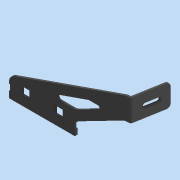
# Autodesk Inventor part: 0 零件
Saved by Autodesk Inventor 2020 (Build 240168000, 168)
## iProperties
Created: 2020-11-03
Part Number: 0 零件
Material: 鋼、碳鋼
Document SubType Name: Sheet Metal
Designer: p2013
Density: 7.85 g/cm^3
Appearance: 一般
Sheet Metal Rule: 預設 mm (_M)
Flat Pattern Width: 7.87536 cm
Flat Pattern Length: 32.1122 cm
Flat Pattern Area: 252.896 cm^2
Sheet Metal Width: 78.754 mm
Sheet Metal Length: 321.122 mm
Sheet Metal Area: 25289.554 mm^2
Author: p2013
Autodesk Inventor part; units mm, degrees
ref_plane "YZ Plane" through (0, 0, 0) normal (1, 0, 0) x (0, 1, 0)
ref_plane "XZ Plane" through (0, 0, 0) normal (0, 1, 0) x (-1, 0, 0)
ref_plane "XY Plane" through (0, 0, 0) normal (0, 0, 1) x (1, 0, 0)
sketch "草圖1" plane through (0, 0, 0) normal (0, 0, 1) x (1, 0, 0)
  line L0 (0, 0) -> (-7.8042, 0) construction
  line L1 (0, 0) -> (0, -16.694) construction
  line L2 (0, 2) -> (0, 12.5)
  line L3 (234.1969, 118.5697) -> (234.1969, 75.5697)
  line L4 (130, 19.7875) -> (130, 12.5) construction
  line L5 (128, 0) -> (2, 0)
  line L6 (234.1969, 118.5697) -> (292.1969, 118.5697)
  line L7 (299.1969, 111.5697) -> (299.1969, 82.5697)
  line L8 (292.1969, 75.5697) -> (234.1969, 75.5697)
  line L9 (256.1969, 101.0697) -> (278.1969, 101.0697)
  arc A0 (278.1969, 93.0697) -> (278.1969, 101.0697) centre (278.1969, 97.0697) ccw
  line L10 (278.1969, 93.0697) -> (256.1969, 93.0697)
  arc A1 (256.1969, 101.0697) -> (256.1969, 93.0697) centre (256.1969, 97.0697) ccw
  line L11 (65, 14) -> (65, 14) construction
  arc A2 (10.0615, 42.1637) -> (0, 28) centre (15, 28) ccw
  line L12 (10.0615, 42.1637) -> (225.9989, 117.4547)
  line L13 (232.5836, 118.5697) -> (234.1969, 118.5697)
  line L14 (234.1969, 75.5697) -> (231.4192, 75.5697)
  line L15 (222.2704, 73.3545) -> (135.4256, 28.6799)
  arc A3 (299.1969, 111.5697) -> (292.1969, 118.5697) centre (292.1969, 111.5697) ccw
  arc A4 (292.1969, 75.5697) -> (299.1969, 82.5697) centre (292.1969, 82.5697) ccw
  arc A5 (135.4256, 28.6799) -> (131.18, 24.5) centre (140, 19.7875) ccw
  line L16 (25.9, 33) -> (39.1, 33)
  line L17 (40.1, 32) -> (40.1, 19)
  line L18 (39.1, 18) -> (25.9, 18)
  line L19 (24.9, 19) -> (24.9, 32)
  line L20 (90.9, 33) -> (104.1, 33)
  line L21 (105.1, 32) -> (105.1, 19)
  line L22 (104.1, 18) -> (90.9, 18)
  line L23 (89.9, 19) -> (89.9, 32)
  line L24 (40.1, 25.5) -> (89.9, 25.5) construction
  line L25 (0, 24.5) -> (2, 24.5)
  line L26 (2, 24.5) -> (2, 12.5)
  line L27 (2, 12.5) -> (0, 12.5)
  line L28 (0, 12.5) -> (0, 24.5) construction
  line L29 (65, 0) -> (65, 25.5) construction
  line L30 (131.18, 24.5) -> (128, 24.5)
  line L31 (128, 24.5) -> (128, 12.5)
  line L32 (128, 12.5) -> (130, 12.5)
  line L33 (130, 12.5) -> (130, 19.7875) construction
  arc A6 (0, 2) -> (2, 0) centre (2, 2) ccw
  arc A7 (128, 0) -> (130, 2) centre (128, 2) ccw
  line L34 (0, 12.5) -> (0, 24.5) construction
  line L35 (0, 24.5) -> (0, 28)
  line L36 (130, 19.7875) -> (130, 24.5) construction
  line L37 (130, 12.5) -> (130, 2)
  line L38 (123.9345, 45) -> (99.3585, 45)
  line L39 (157.566, 75) -> (173.8509, 75)
  line L40 (97.7123, 54.7212) -> (154.2737, 74.4425)
  line L41 (175.452, 68.3877) -> (135.3705, 47.769)
  arc A8 (175.452, 68.3877) -> (173.8509, 75) centre (173.8509, 71.5) ccw
  arc A9 (97.7123, 54.7212) -> (99.3585, 45) centre (99.3585, 50) ccw
  arc A10 (123.9345, 45) -> (135.3705, 47.769) centre (123.9345, 70) ccw
  arc A11 (157.566, 75) -> (154.2737, 74.4425) centre (157.566, 65) ccw
  line L42 (219.0826, 147.5779) -> (251.7371, 53.9233) construction
  arc A12 (232.5836, 118.5697) -> (225.9989, 117.4547) centre (232.5836, 98.5697) ccw
  arc A13 (231.4192, 75.5697) -> (222.2704, 73.3545) centre (231.4192, 55.5697) ccw
  arc A14 (25.9, 33) -> (24.9, 32) centre (25.9, 32) ccw
  arc A15 (40.1, 32) -> (39.1, 33) centre (39.1, 32) ccw
  arc A16 (39.1, 18) -> (40.1, 19) centre (39.1, 19) ccw
  arc A17 (24.9, 19) -> (25.9, 18) centre (25.9, 19) ccw
  arc A18 (89.9, 19) -> (90.9, 18) centre (90.9, 19) ccw
  arc A19 (104.1, 18) -> (105.1, 19) centre (104.1, 19) ccw
  arc A20 (105.1, 32) -> (104.1, 33) centre (104.1, 32) ccw
  arc A21 (90.9, 33) -> (89.9, 32) centre (90.9, 32) ccw
  arc A22 (131.18, 24.5) -> (130, 19.7875) centre (140, 19.7875) ccw construction
  point P0 (130, 0)
  point P1 (299.1969, 118.5697)
  point P2 (299.1969, 75.5697)
  point P3 (130, 25.8889)
  point P4 (229.1969, 118.5697)
  point P5 (24.9, 33)
  point P6 (40.1, 18)
  point P7 (40.1, 33)
  point P8 (24.9, 18)
  point P9 (89.9, 33)
  point P10 (105.1, 18)
  point P11 (105.1, 33)
  point P12 (89.9, 18)
  point P13 (32.5, 33)
  point P14 (97.5, 33)
  point P15 (0, 10.2)
  point P16 (130, 28)
  point P17 (130, 10.2)
  dimension "d0" = 130
  dimension "d2" = 43
  dimension "d3" = 65
  dimension "d4" = 8
  dimension "d5" = 30
  dimension "d7" = 18
  dimension "d14" = 14
  dimension "d17" = 21.5
  dimension "d20" = 15
  dimension "d21" = 28
  dimension "d23" = 5
  dimension "d24" = 7
  dimension "d32" = 10
  dimension "d33" = 8
  dimension "d34" = 15.2
  dimension "d35" = 15.2
  dimension "d36" = 15
  dimension "d37" = 65
  dimension "d38" = 33
  dimension "d39" = 12
  dimension "d40" = 2
  dimension "d41" = 12.5
  dimension "d42" = 2
  dimension "d45" = 45
  dimension "d46" = 17
  dimension "d47" = 17
  dimension "d48" = 30
  dimension "d49" = 3.5
  dimension "d50" = 5
  dimension "d51" = 25
  dimension "d52" = 10
  dimension "d57" = 4.7213
  dimension "d58" = 132.7034
  dimension "d59" = 19.7875
  dimension "d60" = 19.222
  dimension "d61" = 20
  dimension "d62" = 20
  dimension "d63" = 1
  constraints: 87 end point, 53 tangent, 47 point on circle, 32 point on line, 23 centre point, 18 parallel, 11 horizontal, 9 equal radius, 8 perpendicular, 7 midpoint, 5 symmetric about line, 5 vertical, 3 vertical alignment, 2 collinear, 1 coincident
  measures "d0" distance between parallel lines of L4 L2
  measures "d2" distance between parallel lines of L6 L8
  measures "d3" distance between parallel lines of L7 L3
  measures "d4" distance between parallel lines of L10 L9
  measures "d7" distance edge to line of A1 L3
  measures "d14" distance from line of L5 L11.start
  measures "d17" distance from line of L6 A0.centre
  measures "d20" radius of A2
  measures "d21" distance of L0.start L35.end
  measures "d23" distance of point (229.197, 118.57) L3.start
  measures "d24" radius of A3
  measures "d32" radius of A5
  measures "d33" angle of L15 L12
  measures "d34" distance between parallel lines of L17 L19
  measures "d35" distance between parallel lines of L21 L23
  measures "d36" distance between parallel lines of L16 L18
  measures "d37" distance of point (32.5, 33) point (97.5, 33)
  measures "d38" distance between parallel lines of L5 L16
  measures "d39" distance between parallel lines of L27 L25
  measures "d40" distance between parallel lines of L28 L26
  measures "d41" distance between parallel lines of L27 L5
  measures "d42" radius of A6
  measures "d45" distance between parallel lines of L5 L38
  measures "d46" distance between parallel lines of L12 L40
  measures "d47" distance between parallel lines of L15 L41
  measures "d48" distance between parallel lines of L38 L39
  measures "d49" radius of A8
  measures "d50" radius of A9
  measures "d51" radius of A10
  measures "d52" radius of A11
  measures "d57" distance from line of L3.start L42
  measures "d58" distance from line of point (130, 0) L42
  measures "d59" distance from line of L5 A5.centre
  measures "d60" angle of L5 L12
  measures "d61" radius of A12
  measures "d62" radius of A13
  measures "d63" radius of A14
extrude "擠出1" add sketch "草圖1" along normal blind 3.5
bend part "折彎零件1" radius 0.5 angle 80 line through (234.1969, 118.5697, 0) along (0, -1, 0) centre toward (0, 0, -1) moving side (1, 0, 0) both sides no
ref_plane "工作平面1" through (65, 2, 0) normal (-1, 0, 0) x (0, 0, 1)
